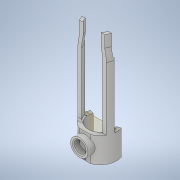
# Autodesk Inventor part: head_adjustable_v5
Saved by Autodesk Inventor 2022 (Build 260153000, 153)
## iProperties
Created: 2018-12-11
Part Number: head_adjustable_v5
Material: Generic
Document SubType Name: Modeling
Designer: Daniel
Density: 1 g/cm^3
Appearance: Default
Author: Daniel
Autodesk Inventor part; units mm, degrees
ref_plane "XZ Plane" through (0, 0, 0) normal (0, 1, 0) x (-1, 0, 0)
sketch "Sketch4" plane through (0, 0, 0) normal (0, 1, 0) x (-1, 0, 0)
  circle A0 centre (0, 0) radius 5.2
  circle A1 centre (0, 0) radius 7
  dimension "d11" = 10.4
  dimension "d12" = 1.8
  constraints: 2 centre point, 2 coincident
  measures "d11" diameter of A0
  measures "d12" radial gap between concentric circles of A1 A0
extrude "Extrusion2" add sketch "Sketch4" along normal blind 10.8
sketch "Sketch16" plane through (0, 10.8, 0) normal (0, 1, 0) x (1, 0, 0)
  circle A0 centre (0, 0) radius 5.2 construction
  circle A1 centre (0, 0) radius 7 construction
  line L0 (-5.3619, -4.5) -> (5.3619, -4.5) construction
  circle A2 centre (0, 0) radius 7 construction
  line L1 (6.9821, 0.5) -> (-6.9821, 0.5) construction
  line L2 (-6.9821, 0.5) -> (-5.1759, 0.5)
  line L3 (-5.3619, -4.5) -> (-2.6058, -4.5)
  circle A3 centre (0, 0) radius 7 construction
  arc A4 (-6.9821, 0.5) -> (-5.3619, -4.5) centre (0, 0) ccw
  arc A5 (-3.4986, -4.5) -> (-3.8067, -4.2425) centre (0, 0) ccw
  line L4 (-4.0643, -4.5) -> (-3.8067, -4.2425)
  point P0 (-3.4986, -4.5)
  point P1 (-5.678, 0.5)
  dimension "d183" = 10.4
  dimension "d131" = 0.5
  dimension "d132" = 4.5
  dimension "d202" = 0.5
  dimension "d207" = 135
  dimension "d208" = 0.4
  constraints: 10 end point, 5 point on circle, 4 point on line, 2 centre point, 2 coincident, 1 concentric, 1 horizontal, 1 parallel, 5 other
  measures "d131" distance from line of point (0, 0) L1
  measures "d132" distance from line of point (0, 0) L0
  measures "d207" angle of L0 L4
  measures "d208" distance from line of A5.start L4
ref_plane "Work Plane5" through (-6.9821, 10.8, -0.5) normal (0, 0, 1) x (1, 0, 0)
sketch "Sketch23" plane through (-6.9821, 10.8, -0.5) normal (0, 0, 1) x (1, 0, 0)
  line L0 (0, 0) -> (0, 27)
  line L1 (0, 27) -> (0, 29.9869) construction
  line L2 (0, 29.9869) -> (0.6, 30.3333) construction
  line L3 (0.6, 30.3333) -> (0.6, 32) construction
  spline S0 degree 3 poles (0, 27) (0, 29.9869) (0.6, 30.3333) (0.6, 32) knots 1 1 1 1 2 2 2 2
  line L4 (0.6, 32) -> (0.6, 37)
  point P0 (6.9821, -10.8)
  dimension "d191" = 120
  dimension "d192" = 37
  dimension "d194" = 5
  dimension "d195" = 1.6667
  dimension "d205" = 0.6
  constraints: 4 end point, 4 vertical, 1 coincident, 3 other
  measures "d191" angle of L1 L2
  measures "d192" vertical distance of point (0, 0) L4.end
  measures "d194" vertical distance of L3.end L0.end
  measures "d195" distance of L3.end L2.end
  measures "d205" distance between parallel lines of L0 L4
sweep "Sweep1" add profiles "Sketch16" path "Sketch23" keep normal constant yes contours L2 A5 L4 L3 A4
sketch "Sketch9" plane through (0, 0, 0) normal (1, 0, 0) x (0, 1, 0)
  line L0 (51.7488, 3.5) -> (10, 3.5)
  line L1 (39.3, 1.5) -> (38.8, 1)
  line L2 (51.7488, 3.5) -> (51.7488, 1.5)
  line L3 (38.8, 1) -> (10.8, 1)
  line L4 (10.8, 4.5) -> (10.8, -7) construction
  line L5 (10.8, 4.5) -> (10.8, -7)
  line L6 (10.8, -7) -> (58.7483, -7)
  line L7 (58.7483, -7) -> (58.7483, 7)
  line L8 (58.7483, 7) -> (10.8, 7)
  line L9 (10.8, 1) -> (10.8, 7)
  line L10 (51.7488, 1.5) -> (39.3, 1.5)
  line L11 (0, 7) -> (10.8, 7) construction
  line L12 (0, 5.2) -> (0, 7) construction
  line L13 (10.8, 5.2) -> (0, 5.2) construction
  line L14 (10.8, 7) -> (10.8, 5.2) projected
  line L15 (10.8, -7) -> (0, -7) construction
  line L16 (10.8, -5.2) -> (10.8, -7) projected
  line L17 (0, -5.2) -> (10.8, -5.2) construction
  line L18 (0, -7) -> (0, -5.2) construction
  line L19 (10.8, -0.5) -> (37.8, -0.5) construction
  line L20 (10.8, 4.5) -> (37.8, 4.5) projected
  point P0 (0, 0)
  point P1 (10, 3.5)
  point P2 (10.8, 3.5)
  dimension "d147" = 28
  dimension "d170" = 0.5
  dimension "d203" = 1.5
  dimension "d204" = 135
  dimension "d209" = 2
  constraints: 18 end point, 3 collinear, 3 perpendicular, 3 vertical, 2 horizontal, 7 other
  measures "d147" distance of L1.end L3.end
  measures "d170" distance between parallel lines of L3 L10
  measures "d203" distance between parallel lines of L3 L19
  measures "d204" angle of L3 L1
extrude "Extrusion4" cut sketch "Sketch9" along normal through all both and the other way through all contours L0 L5 L9 L8 L7 L6 L3 L1 L10 L2
ref_plane "Work Plane2" through (-9.1, 0, 0) normal (1, 0, 0) x (0, 1, 0)
mirror "Mirror3" about plane through (0, 0, 0) normal (1, 0, 0) of "Extrusion4", "Sweep1"
sketch "Sketch18" plane through (0, 10.8, 0) normal (0, 1, 0) x (1, 0, 0)
  line L0 (-2.3324, -6.6) -> (2.3324, -6.6)
  circle A0 centre (0, 0) radius 7 projected
  point P0 (0, -7)
  point P1 (0, -7)
  point P2 (6.9282, -1)
  point P3 (-6.9282, -1)
  point P4 (-5.3244, -4.2297)
  point P5 (5.3244, -4.2297)
  dimension "d159" = 0.4
  constraints: 2 end point, 1 horizontal, 3 other
extrude "Extrusion9" cut sketch "Sketch18" against normal through all contours L0 A0 picked at (-0.2636, -6.7184)
sketch "Sketch19" plane through (-2.3324, 10.8, 6.6) normal (0, 0, 1) x (1, 0, 0)
  circle A0 centre (2.3324, -10) radius 0.5
  line L0 (4.6648, -10.8) -> (0, -10.8) projected
  point P0 (2.3324, -10.8)
  point P1 (2.3324, -10.8)
  dimension "d162" = 1
  dimension "d163" = 0.8
  constraints: 1 centre point, 1 midpoint, 1 vertical alignment
  measures "d162" diameter of A0
  measures "d163" distance of point (2.332, -10.8) A0.centre
extrude "Extrusion10" cut sketch "Sketch19" against normal up to next
sketch "Sketch20" plane through (0, 0, 0) normal (0, -1, 0) x (1, 0, 0)
  line L0 (0, 0) -> (18.8941, -6.8769)
  line L1 (18.8941, -6.8769) -> (18.8941, 20.0376)
  line L2 (18.8941, 20.0376) -> (-19.5775, 20.0376)
  line L3 (-19.5775, 20.0376) -> (-19.5775, -7.1256)
  line L4 (-19.5775, -7.1256) -> (0, 0)
  line L5 (18.8941, -6.8769) -> (18.8941, -16.9481)
  line L6 (18.8941, -16.9481) -> (-19.5775, -16.9481)
  line L7 (-19.5775, -16.9481) -> (-19.5775, -7.1256)
  dimension "d166" = 70
  dimension "d167" = 70
  dimension "d172" = 140
  constraints: 16 end point, 4 perpendicular, 2 vertical
  measures "d166" angle of L3 L4
  measures "d167" angle of L1 L0
  measures "d172" angle of L0 L4
extrude "Extrusion11" cut sketch "Sketch20" against normal through all contours L0 L5 L6 L7 L4
sketch "Sketch21" plane through (-2.3324, 10.8, 6.6) normal (0, 0, 1) x (1, 0, 0)
  circle A0 centre (2.3324, -4.8) radius 2.525
  circle A1 centre (2.3324, -4.8) radius 3.725
  line L0 (4.6648, -10.8) -> (0, -10.8) projected
  point P0 (2.3324, -10.8)
  point P1 (2.3324, -10.8)
  dimension "d173" = 5.05
  dimension "d174" = 1.2
  dimension "d175" = 6
  constraints: 2 centre point, 1 midpoint, 1 vertical alignment
  measures "d173" diameter of A0
  measures "d174" radial gap between concentric circles of A0 A1
  measures "d175" distance from line of L0 A0.centre
extrude "Extrusion12" add sketch "Sketch21" against normal up to next
extrude "Extrusion13" add sketch "Sketch21" along normal blind 2.4
chamfer "Chamfer7" distance 0.4 angle 45 1 edges at (-2.525, 6, 9)
fillet "Fillet11" radius 0.6 5 edges at (-5.2805, 10.8, 3.5) (-6.2699, 10.8, 1) (6.2699, 10.8, 1) (-5.2075, 10.8, 2.3178) (5.2075, 10.8, 2.3178)
body "Solid2"
